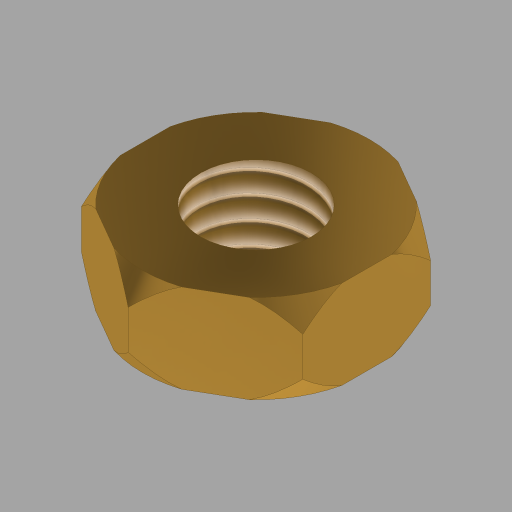
# Autodesk Inventor part: Nut_M2_Brass
Saved by Autodesk Inventor 2024 (Build 280153020, 153B)
## iProperties
Created: 2023-06-05
Part Number: Nut_M2_Brass
Material: Brass
Document SubType Name: Modeling
Designer: schanen
Density: 8.49 g/cm^3
Appearance: Brass - Polished
Author: schanen
Autodesk Inventor part; units mm, degrees
ref_plane "YZ Plane" through (0, 0, 0) normal (1, 0, 0) x (0, 1, 0)
ref_plane "XZ Plane" through (0, 0, 0) normal (0, 1, 0) x (-1, 0, 0)
ref_plane "XY Plane" through (0, 0, 0) normal (0, 0, 1) x (1, 0, 0)
sketch "Sketch1" plane through (0, 0, 0) normal (0, 1, 0) x (-1, 0, 0)
  line L0 (2, 1.1547) -> (2, -1.1547)
  line L1 (2, -1.1547) -> (0, -2.3094)
  line L2 (0, -2.3094) -> (-2, -1.1547)
  line L3 (-2, -1.1547) -> (-2, 1.1547)
  line L4 (-2, 1.1547) -> (0, 2.3094)
  line L5 (0, 2.3094) -> (2, 1.1547)
  circle A0 centre (0, 0) radius 1
  dimension "d0" = 4
  dimension "d1" = 2
  constraints: 12 end point, 2 coincident, 1 centre point, 1 vertical alignment, 13 other
  measures "d0" distance between parallel lines of L3 L0
  measures "d1" diameter of A0
extrude "Extrusion1" add sketch "Sketch1" along normal blind 1.6
thread "Thread1" size "M2x0.4" class "6H" standard "ISO Metric profile" length 11.5
sketch "Sketch2" plane through (0, 1.6, 0) normal (0, 1, 0) x (1, 0, 0)
  circle A0 centre (0, 0) radius 2.05
  dimension "d7" = 4.1
  constraints: 1 centre point, 1 coincident
  measures "d7" diameter of A0
extrude "Extrusion2" cut sketch "Sketch2" against normal blind 1.6 draft 30 keep common part
sketch "Sketch3" plane through (0, 0, 0) normal (0, -1, 0) x (1, 0, 0)
  circle A0 centre (0, 0) radius 2.05
  dimension "d10" = 4.1
  constraints: 1 centre point, 1 coincident
  measures "d10" diameter of A0
extrude "Extrusion3" cut sketch "Sketch3" against normal blind 1.6 draft 30 keep common part
body "Solid1"
